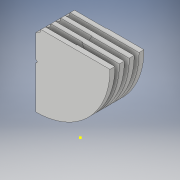
# Autodesk Inventor part: 밑판 메인
Saved by Autodesk Inventor 2019.5 (Build 235369000, 369)
## iProperties
Created: 2021-07-19
Part Number: 밑판 메인
Material: 일반
Document SubType Name: Modeling
Designer: msj19
Density: 1 g/cm^3
Appearance: 기본값
Author: msj19
Autodesk Inventor part; units mm, degrees
note: some values were not read from the file. Chosen so that the rebuilt part matches the saved one: kept side of "분할1".
ref_plane "우측면도" through (0, 0, 0) normal (1, 0, 0) x (0, 1, 0)
ref_plane "평면도" through (0, 0, 0) normal (0, 1, 0) x (-1, 0, 0)
ref_plane "정면도" through (0, 0, 0) normal (0, 0, 1) x (1, 0, 0)
sketch "스케치1" plane through (0, 0, 0) normal (0, 0, 1) x (1, 0, 0)
  line L0 (0, 0) -> (19.5, -32.9882) construction
  circle A0 centre (92, 32.0118) radius 10
  circle A1 centre (143.7697, 61.8433) radius 2.5
  circle A2 centre (40.2303, 61.8433) radius 2.5
  circle A3 centre (92, -28.4882) radius 2.5
  circle A4 centre (92, 32.0118) radius 150
  line L1 (-58, 32.0118) -> (242, 32.0118)
  dimension "d5" = 20
  dimension "d7" = 5
  dimension "d10" = 5
  dimension "d14" = 5
  dimension "d16" = 300
  dimension "d18" = 59.7497
  dimension "d19" = 60.5
  dimension "d20" = 59.7497
  dimension "d21" = 97.4103
  constraints: 5 centre point, 4 end point, 2 point on circle, 1 coincident
  measures "d5" diameter of A0
  measures "d7" diameter of A1
  measures "d10" diameter of A2
  measures "d14" diameter of A3
  measures "d16" diameter of A4
  measures "d18" distance of A0.centre A2.centre
  measures "d19" distance of A3.centre A0.centre
  measures "d20" distance of A1.centre A0.centre
  measures "d21" distance of A0.centre L0.start
extrude "돌출1" add sketch "스케치1" against normal blind 10 contours L1 A4 A0 | A0 L1 A4
sketch "스케치2" plane through (0, 0, 0) normal (0, 0, 1) x (1, 0, 0)
  line L0 (72, 127.0118) -> (0, 0)
  line L1 (184, 0) -> (112, 127.0118)
  line L2 (19.5, -32.9882) -> (164.5, -32.9882)
  line L3 (72, 127.0118) -> (112, 127.0118)
  line L4 (0, 0) -> (19.5, -32.9882)
  line L5 (164.5, -32.9882) -> (184, 0)
  circle A0 centre (92, 32.0118) radius 10
  circle A1 centre (143.7697, 61.8433) radius 2
  circle A2 centre (40.2303, 61.8433) radius 2
  circle A3 centre (92, -28.4882) radius 2
  dimension "d24" = 184
  dimension "d25" = 146
  dimension "d26" = 146
  dimension "d27" = 145
  dimension "d28" = 40
  dimension "d29" = 20
  dimension "d30" = 65
  dimension "d31" = 4
  dimension "d32" = 4.5
  dimension "d33" = 72.5
  dimension "d34" = 4
  dimension "d35" = 4.5
  dimension "d36" = 72.5
  dimension "d37" = 4.5
  dimension "d38" = 4
  dimension "d39" = 72.5
  constraints: 12 end point, 4 centre point, 2 horizontal, 1 point on line
  measures "d24" distance of L0.end L1.start
  measures "d25" distance of L0.start L0.end
  measures "d26" distance of L1.end L1.start
  measures "d27" distance of L2.start L2.end
  measures "d28" distance of L0.start L1.end
  measures "d29" diameter of A0
  measures "d30" distance from line of L2 A0.centre
  measures "d31" diameter of A1
  measures "d32" distance from line of L1 A1.centre
  measures "d33" distance of A1.centre L1.end
  measures "d34" diameter of A2
  measures "d35" distance from line of L0 A2.centre
  measures "d36" distance of A2.centre L0.start
  measures "d37" distance from line of L2 A3.centre
  measures "d38" diameter of A3
  measures "d39" horizontal distance of A3.centre L2.start
extrude "돌출2" cut sketch "스케치2" against normal blind 1
sketch "스케치3" plane through (92, 32.0118, 0) normal (0, 0, 1) x (1, 0, 0)
  line L0 (0, 195.8297) -> (0, -216.3238)
  point P0 (-92, -32.0118)
  constraints: 2 end point
surface extrude "돌출 곡면1" sketch "스케치3" along normal mid plane 739.5 shown no curves L0
sketch "스케치4" plane through (0, 0, 0) normal (0, 0, 1) x (1, 0, 0)
  line L0 (-58, 32.0118) -> (242, 32.0118)
  point P0 (0, 0)
  constraints: 2 end point
sketch "스케치5" plane through (0, 0, -1) normal (0, 0, 1) x (1, 0, 0)
  point P0 (0, 0)
surface extrude "돌출 곡면2" sketch "스케치4" along normal mid plane 739.5 shown no curves L0
split body "분할1" result two bodies by surface "돌출 곡면2" first body at (45.9032, -16.1061, -9.5)
split body "분할2" result two bodies by surface "돌출 곡면1" bodies 3 first body at (108.6328, 95.8416, -9.5)
split body "분할3" result two bodies by surface "돌출 곡면1" bodies 2 first body at (138.1519, -16.0173, -9.5)
move or copy body "본체 이동1" bodies to move or copy 6 copy no translate (-150, 150, 12)
move or copy body "본체 이동2" bodies to move or copy 4 copy no translate (-150, 0, -12)
move or copy body "본체 이동3" bodies to move or copy 7 copy no translate (0, 150, 24)
move or copy body "본체 이동4" bodies to move or copy 7 copy no translate (0, 0, 3)
move or copy body "본체 이동5" bodies to move or copy 4 copy no translate (0, 0, 6)
move or copy body "본체 이동6" bodies to move or copy 4 copy no translate (0, 0, -12)
move or copy body "본체 이동7" bodies to move or copy 5 copy no translate (0, 0, -6)
move or copy body "본체 이동8" bodies to move or copy 5 copy no translate (0, 0, 3)
move or copy body "본체 이동9" bodies to move or copy 7 copy no rotation origin (0, 0, 0) rotation axis (0, 1, 0) rotation angle 180 translate (184, 0, 54)
move or copy body "본체 이동10" bodies to move or copy 4 copy no rotation origin (0, 0, 0) rotation axis (1, 0, 0) rotation angle -180 translate (0, 64.0236, -56)
move or copy body "본체 이동11" bodies to move or copy 5 copy no rotation origin (0, 0, 0) rotation axis (0, 1, 0) rotation angle -180 translate (184, 0, -26)
move or copy body "본체 이동12" bodies to move or copy 5 copy no rotation origin (0, 0, 0) rotation axis (1, 0, 0) rotation angle -180 translate (0, 64.0236, -46)
move or copy body "본체 이동13" bodies to move or copy 7 copy no translate (-150, 0, 0)
move or copy body "본체 이동14" bodies to move or copy 5 copy no translate (-150, 150, 0)
move or copy body "본체 이동15" bodies to move or copy 4 copy no translate (0, 150, 0)
move or copy body "본체 이동16" bodies to move or copy 5 copy no translate (0, 0, 12)
move or copy body "본체 이동17" bodies to move or copy 7 copy no translate (0, 0, -6)
move or copy body "본체 이동18" bodies to move or copy 5 copy no translate (0, 0, 3)
body "Srf1"
body "Srf2"
